Autodesk Inventor part; units mm, degrees
(part 6 of 9)
sketch "Sketch39" plane through (0, 0, 0) normal (1, 0, 0) x (0, 0, -1)
  line L0 (-85.3603, 16.259) -> (-85.3603, 6.734)
  arc A0 (-90.1228, 1.9715) -> (-85.3603, 6.734) centre (-90.1228, 6.734) ccw
  line L1 (-90.1228, 1.9715) -> (-121.8728, 1.9715)
  arc A1 (-126.6353, 6.734) -> (-121.8728, 1.9715) centre (-121.8728, 6.734) ccw
  line L2 (-126.6353, 6.734) -> (-126.6353, 16.259)
  line L3 (-126.6353, 16.259) -> (-132.3503, 16.259)
  arc A2 (-132.3503, 22.609) -> (-132.3503, 16.259) centre (-132.3503, 19.434) ccw
  line L4 (-132.3503, 22.609) -> (-126.6353, 22.609)
  line L5 (-126.6353, 22.609) -> (-126.6353, 32.134)
  arc A3 (-121.8728, 36.8965) -> (-126.6353, 32.134) centre (-121.8728, 32.134) ccw
  line L6 (-121.8728, 36.8965) -> (-90.1228, 36.8965)
  arc A4 (-85.3603, 32.134) -> (-90.1228, 36.8965) centre (-90.1228, 32.134) ccw
  line L7 (-85.3603, 32.134) -> (-85.3603, 22.609)
  line L8 (-85.3603, 22.609) -> (-79.6453, 22.609)
  arc A5 (-79.6453, 16.259) -> (-79.6453, 22.609) centre (-79.6453, 19.434) ccw
  line L9 (-79.6453, 16.259) -> (-85.3603, 16.259)
  line L10 (-121.8728, 6.734) -> (-90.1228, 6.734)
  line L11 (-90.1228, 6.734) -> (-90.1228, 32.134)
  line L12 (-90.1228, 32.134) -> (-121.8728, 32.134)
  line L13 (-121.8728, 32.134) -> (-121.8728, 6.734)
  line L14 (-121.8728, 6.734) -> (-90.1228, 32.134) construction
  line L15 (-90.1228, 6.734) -> (-121.8728, 32.134) construction
  line L16 (-131.3978, 57.3308) -> (-80.5978, 57.3308)
  line L17 (-105.9978, 19.434) -> (-105.9978, 57.3308)
  line L18 (-105.9978, -16.3292) -> (-105.9978, 19.434)
  line L19 (-112.3478, -16.3292) -> (-99.6478, -16.3292)
  circle A6 centre (-112.3478, -16.3292) radius 2.5527
  circle A7 centre (-99.6478, -16.3292) radius 2.5527
  circle A8 centre (-80.5978, 57.3308) radius 2.5527
  circle A9 centre (-131.3978, 57.3308) radius 2.5527
  line L20 (-112.3478, -13.7765) -> (-99.6478, -13.7765)
  line L21 (-99.6478, -18.8819) -> (-112.3478, -18.8819)
  line L22 (-131.3978, 59.8835) -> (-80.5978, 59.8835)
  line L23 (-80.5978, 54.7781) -> (-131.3978, 54.7781)
  arc A10 (-196.307, 76.2) -> (-199.482, 73.025) centre (-196.307, 73.025) ccw projected
  line L24 (-199.482, 73.025) -> (-199.482, -252.424) projected
  arc A11 (-199.482, -252.424) -> (-196.307, -255.599) centre (-196.307, -252.424) ccw projected
  line L25 (-196.307, -255.599) -> (147.8383, -255.599) projected
  arc A12 (147.8383, -255.599) -> (150.6952, -253.8092) centre (147.8383, -252.424) ccw projected
  line L26 (194.4526, -163.563) -> (150.6952, -253.8092) projected
  arc A13 (194.8736, -162.9119) -> (194.4526, -163.563) centre (197.3095, -164.9483) ccw projected
  arc A14 (194.8736, -162.9119) -> (235.5329, 95.0804) centre (0, 0) ccw projected
  arc A15 (235.5329, 95.0804) -> (218.389, 101.8364) centre (223.7562, 90.3263) ccw projected
  line L27 (218.389, 101.8364) -> (173.6183, 80.9596) projected
  arc A16 (152.1493, 76.2) -> (173.6183, 80.9596) centre (152.1493, 127) ccw projected
  line L28 (152.1493, 76.2) -> (-196.307, 76.2) projected
  arc A17 (-166.8187, -7.1514) -> (-170.0188, -10.965) centre (-168.4187, -9.0582) ccw projected
  arc A18 (-166.8187, -7.1514) -> (-135.2171, -21.8874) centre (-123.52, 44.45) ccw projected
  arc A19 (-136.0816, -26.7902) -> (-135.2171, -21.8874) centre (-135.6494, -24.3388) ccw projected
  arc A20 (-170.0188, -10.965) -> (-136.0816, -26.7902) centre (-123.52, 44.45) ccw projected
  circle A21 centre (-123.52, 44.45) radius 2.4892 projected
  line L29 (-117.9165, 59.8835) -> (-80.5978, 59.8835) projected
  arc A22 (-80.5978, 54.7781) -> (-80.5978, 59.8835) centre (-80.5978, 57.3308) ccw projected
  line L30 (-80.5978, 54.7781) -> (-123.0219, 54.7781) projected
  line L31 (-123.0219, 54.7781) -> (-117.9165, 59.8835) projected
  circle A23 centre (-11.1125, -19.2474) radius 2.2479 projected
  circle A24 centre (-11.1125, 19.2474) radius 2.2479 projected
  circle A25 centre (22.225, 0) radius 2.2479 projected
  circle A26 centre (11.1125, 19.2474) radius 2.2479 projected
  circle A27 centre (-22.225, 0) radius 2.2479 projected
  circle A28 centre (11.1125, -19.2474) radius 2.2479 projected
  line L32 (-112.3478, -13.7765) -> (-99.6478, -13.7765) projected
  arc A29 (-99.6478, -18.8819) -> (-99.6478, -13.7765) centre (-99.6478, -16.3292) ccw projected
  line L33 (-99.6478, -18.8819) -> (-112.3478, -18.8819) projected
  arc A30 (-112.3478, -13.7765) -> (-112.3478, -18.8819) centre (-112.3478, -16.3292) ccw projected
  circle A31 centre (-58.8554, 19.434) radius 2.4892 projected
  circle A32 centre (-76.4174, -178.6042) radius 13.335 projected
  circle A33 centre (-187.1176, -166.8269) radius 2.4892 projected
  circle A34 centre (-174.2102, -166.8866) radius 2.4892 projected
  circle A35 centre (-167.2175, -120.5501) radius 2.4892 projected
  circle A36 centre (-180.1195, -116.9252) radius 2.4892 projected
  circle A37 centre (-193.0957, -120.1058) radius 2.4892 projected
  circle A38 centre (-186.8225, -117.6771) radius 2.4892 projected
  circle A39 centre (-173.4354, -117.9041) radius 2.4892 projected
  circle A40 centre (-168.1768, -164.3742) radius 2.4892 projected
  circle A41 centre (-180.6733, -167.7222) radius 2.4892 projected
  circle A42 centre (-193.0957, -164.2646) radius 2.4892 projected
  arc A43 (-177.4857, -133.2108) -> (-183.7867, -151.2692) centre (-180.6362, -142.24) ccw projected
  arc A44 (-183.3071, -151.4366) -> (-177.0061, -133.3781) centre (-180.1566, -142.4074) ccw projected
  circle A45 centre (-85.7798, -94.9817) radius 2.4892 projected
  circle A46 centre (-110.3931, -99.2933) radius 2.4892 projected
  circle A47 centre (-101.8395, -50.0579) radius 2.4892 projected
  circle A48 centre (-124.2369, -62.8574) radius 2.4892 projected
  circle A49 centre (-110.6604, -51.6228) radius 2.4892 projected
  circle A50 centre (-93.2858, -99.3592) radius 2.4892 projected
  circle A51 centre (-116.932, -39.699) radius 2.5527 projected
  circle A52 centre (-118.4334, -56.0666) radius 2.4892 projected
  circle A53 centre (-93.0185, -51.5569) radius 2.4892 projected
  circle A54 centre (-101.8395, -100.8579) radius 2.4892 projected
  circle A55 centre (-80.2428, -88.2574) radius 2.4892 projected
  arc A56 (-99.4903, -84.728) -> (-104.0551, -66.155) centre (-101.7058, -75.4251) ccw projected
  arc A57 (-99.6119, -84.758) -> (-99.4903, -84.728) centre (-101.8395, -75.4579) ccw projected
  arc A58 (-99.7334, -84.7881) -> (-99.6119, -84.758) centre (-101.9731, -75.491) ccw projected
  arc A59 (-99.8547, -84.8183) -> (-99.7334, -84.7881) centre (-102.1066, -75.5241) ccw projected
  arc A60 (-104.4917, -66.2632) -> (-99.8547, -84.8183) centre (-102.2399, -75.5574) ccw projected
  arc A61 (-104.3463, -66.227) -> (-104.4917, -66.2632) centre (-102.1066, -75.5241) ccw projected
  arc A62 (-104.2008, -66.1909) -> (-104.3463, -66.227) centre (-101.9731, -75.491) ccw projected
  arc A63 (-104.0551, -66.155) -> (-104.2008, -66.1909) centre (-101.8395, -75.4579) ccw projected
  circle A64 centre (239.2356, -31.496) radius 3.3782 projected
  circle A65 centre (223.7295, 90.3926) radius 3.3782 projected
  circle A66 centre (239.2356, 31.496) radius 3.3782 projected
  circle A67 centre (221.404, -95.9477) radius 3.3782 projected
  line L34 (149.831, -89.2272) -> (89.9434, -38.9755) projected
  arc A68 (88.9, -36.7379) -> (89.9434, -38.9755) centre (91.821, -36.7379) ccw projected
  line L35 (88.9, -36.7379) -> (88.9, -15.621) projected
  arc A69 (91.821, -12.7) -> (88.9, -15.621) centre (91.821, -15.621) ccw projected
  line L36 (91.821, -12.7) -> (174.1799, -12.7) projected
  arc A70 (177.0893, -15.8819) -> (174.1799, -12.7) centre (174.1799, -15.621) ccw projected
  arc A71 (154.2425, -88.4425) -> (177.0893, -15.8819) centre (0, 0) ccw projected
  arc A72 (149.831, -89.2272) -> (154.2425, -88.4425) centre (151.7086, -86.9895) ccw projected
  line L37 (88.9, -0.254) -> (88.9, 0.254) projected
  arc A73 (91.821, 3.175) -> (88.9, 0.254) centre (91.821, 0.254) ccw projected
  line L38 (91.821, 3.175) -> (174.4218, 3.175) projected
  arc A74 (177.3428, 0.254) -> (174.4218, 3.175) centre (174.4218, 0.254) ccw projected
  line L39 (177.3428, 0.254) -> (177.3428, -0.254) projected
  arc A75 (174.4218, -3.175) -> (177.3428, -0.254) centre (174.4218, -0.254) ccw projected
  line L40 (174.4218, -3.175) -> (91.821, -3.175) projected
  arc A76 (88.9, -0.254) -> (91.821, -3.175) centre (91.821, -0.254) ccw projected
  arc A77 (177.0893, 15.8819) -> (169.6939, 53.0738) centre (0, 0) ccw projected
  arc A78 (174.1799, 12.7) -> (177.0893, 15.8819) centre (174.1799, 15.621) ccw projected
  line L41 (174.1799, 12.7) -> (91.821, 12.7) projected
  arc A79 (88.9, 15.621) -> (91.821, 12.7) centre (91.821, 15.621) ccw projected
  line L42 (88.9, 15.621) -> (88.9, 17.1891) projected
  arc A80 (90.5865, 19.8364) -> (88.9, 17.1891) centre (91.821, 17.1891) ccw projected
  line L43 (90.5865, 19.8364) -> (165.6716, 54.8492) projected
  arc A81 (169.6939, 53.0738) -> (165.6716, 54.8492) centre (166.9061, 52.2019) ccw projected
  arc A82 (180.8991, -105.7674) -> (203.0448, 51.8076) centre (0, 0) ccw projected
  arc A83 (204.8485, 54.889) -> (203.0448, 51.8076) centre (205.5059, 52.4355) ccw projected
  line L44 (204.8485, 54.889) -> (206.0753, 55.2177) projected
  arc A84 (209.1938, 53.3924) -> (206.0753, 55.2177) centre (206.7327, 52.7643) ccw projected
  arc A85 (186.3731, -108.9857) -> (209.1938, 53.3924) centre (0, 0) ccw projected
  arc A86 (182.8723, -109.8807) -> (186.3731, -108.9857) centre (184.1805, -107.7035) ccw projected
  line L45 (182.8723, -109.8807) -> (181.7836, -109.2266) projected
  arc A87 (180.8991, -105.7674) -> (181.7836, -109.2266) centre (183.0918, -107.0494) ccw projected
  arc A88 (159.1231, -92.6879) -> (178.5072, 45.237) centre (0, 0) ccw projected
  arc A89 (180.312, 48.3145) -> (178.5072, 45.237) centre (180.9694, 45.861) ccw projected
  line L46 (180.312, 48.3145) -> (181.5388, 48.6432) projected
  arc A90 (184.6584, 46.8139) -> (181.5388, 48.6432) centre (182.1962, 46.1897) ccw projected
  arc A91 (164.6013, -95.8992) -> (184.6584, 46.8139) centre (0, 0) ccw projected
  arc A92 (161.0985, -96.7977) -> (164.6013, -95.8992) centre (162.4067, -94.6205) ccw projected
  line L47 (161.0985, -96.7977) -> (160.0098, -96.1436) projected
  arc A93 (159.1231, -92.6879) -> (160.0098, -96.1436) centre (161.3179, -93.9664) ccw projected
  line L48 (171.9854, -103.3393) -> (170.8967, -102.6851) projected
  arc A94 (170.0112, -99.2275) -> (170.8967, -102.6851) centre (172.2049, -100.5079) ccw projected
  arc A95 (170.0112, -99.2275) -> (190.7761, 48.5222) centre (0, 0) ccw projected
  arc A96 (192.5803, 51.6017) -> (190.7761, 48.5222) centre (193.2377, 49.1483) ccw projected
  line L49 (192.5803, 51.6017) -> (193.8071, 51.9305) projected
  arc A97 (196.9261, 50.1033) -> (193.8071, 51.9305) centre (194.4645, 49.477) ccw projected
  arc A98 (175.4872, -102.4426) -> (196.9261, 50.1033) centre (0, 0) ccw projected
  arc A99 (171.9854, -103.3393) -> (175.4872, -102.4426) centre (173.2936, -101.1621) ccw projected
  circle A100 centre (187.962, 68.4126) radius 2.5527 projected
  circle A101 centre (0, 0) radius 13.335 projected
  circle A102 centre (160.7915, -118.9794) radius 2.5527 projected
  circle A103 centre (145.0649, -113.4346) radius 2.5527 projected
  circle A104 centre (122.2368, -242.899) radius 2.5527 projected
  circle A105 centre (70.3186, -242.899) radius 2.5527 projected
  circle A106 centre (97.9437, -242.899) radius 2.5527 projected
  circle A107 centre (145.0649, -242.899) radius 2.5527 projected
  circle A108 centre (-116.932, -242.899) radius 2.5527 projected
  circle A109 centre (-116.932, -179.399) radius 2.5527 projected
  circle A110 centre (-148.682, -179.399) radius 2.5527 projected
  circle A111 centre (-186.782, -39.699) radius 2.5527 projected
  circle A112 centre (-186.782, -242.899) radius 2.5527 projected
  circle A113 centre (67.218, 63.5) radius 2.5527 projected
  circle A114 centre (-59.782, 63.5) radius 2.5527 projected
  circle A115 centre (-8.982, 63.5) radius 2.5527 projected
  circle A116 centre (143.418, 63.5) radius 2.5527 projected
  circle A117 centre (-186.782, -179.399) radius 2.5527 projected
  circle A118 centre (-148.682, -39.699) radius 2.5527 projected
  circle A119 centre (-148.682, -242.899) radius 2.5527 projected
  arc A120 (-82.1853, 16.259) -> (-85.3603, 13.084) centre (-82.1853, 13.084) ccw projected
  line L50 (-85.3603, 13.084) -> (-85.3603, 6.734) projected
  arc A121 (-90.1228, 1.9715) -> (-85.3603, 6.734) centre (-90.1228, 6.734) ccw projected
  line L51 (-90.1228, 1.9715) -> (-121.8728, 1.9715) projected
  arc A122 (-126.6353, 6.734) -> (-121.8728, 1.9715) centre (-121.8728, 6.734) ccw projected
  line L52 (-126.6353, 6.734) -> (-126.6353, 13.084) projected
  arc A123 (-126.6353, 13.084) -> (-129.8103, 16.259) centre (-129.8103, 13.084) ccw projected
  line L53 (-129.8103, 16.259) -> (-132.3503, 16.259) projected
  arc A124 (-132.3503, 22.609) -> (-132.3503, 16.259) centre (-132.3503, 19.434) ccw projected
  line L54 (-132.3503, 22.609) -> (-129.8103, 22.609) projected
  arc A125 (-129.8103, 22.609) -> (-126.6353, 25.784) centre (-129.8103, 25.784) ccw projected
  line L55 (-126.6353, 25.784) -> (-126.6353, 32.134) projected
  arc A126 (-121.8728, 36.8965) -> (-126.6353, 32.134) centre (-121.8728, 32.134) ccw projected
  line L56 (-121.8728, 36.8965) -> (-90.1228, 36.8965) projected
  arc A127 (-85.3603, 32.134) -> (-90.1228, 36.8965) centre (-90.1228, 32.134) ccw projected
  line L57 (-85.3603, 32.134) -> (-85.3603, 25.784) projected
  arc A128 (-85.3603, 25.784) -> (-82.1853, 22.609) centre (-82.1853, 25.784) ccw projected
  line L58 (-82.1853, 22.609) -> (-79.6453, 22.609) projected
  arc A129 (-79.6453, 16.259) -> (-79.6453, 22.609) centre (-79.6453, 19.434) ccw projected
  line L59 (-79.6453, 16.259) -> (-82.1853, 16.259) projected
  line L60 (-121.8728, 32.134) -> (-90.1228, 6.734)
  line L61 (-90.1228, 32.134) -> (-121.8728, 6.734)
  arc A130 (-90.1228, 1.9715) -> (-85.3603, 6.734) centre (-90.1228, 6.734) ccw projected
  line L62 (-121.8728, 36.8965) -> (-90.1228, 36.8965) projected
  line L63 (-85.3603, 32.134) -> (-85.3603, 25.784) projected
  line L64 (-126.6353, 6.734) -> (-126.6353, 13.084) projected
  arc A131 (-85.3603, 32.134) -> (-90.1228, 36.8965) centre (-90.1228, 32.134) ccw projected
  arc A132 (-132.3503, 22.609) -> (-132.3503, 16.259) centre (-132.3503, 19.434) ccw projected
  line L65 (-132.3503, 22.609) -> (-129.8103, 22.609) projected
  line L66 (-129.8103, 16.259) -> (-132.3503, 16.259) projected
  line L67 (-177.4857, -133.2108) -> (-177.0061, -133.3781) projected
  line L68 (-183.3071, -151.4366) -> (-183.7867, -151.2692) projected
  point P0 (-105.9978, 19.434)
  dimension "d863" = 50.8
  dimension "d864" = 12.7
  dimension "d865" = 5.1054
  dimension "d866" = 35.7632
  dimension "d867" = 37.8968
  constraints: 52 end point, 21 point on circle, 10 centre point, 10 coincident, 10 collinear, 10 equal radius, 10 midpoint, 7 tangent, 4 horizontal, 2 parallel, 2 point on line, 2 vertical, 1 perpendicular
  measures "d863" distance of L16.end L16.start
  measures "d864" distance of L19.start L19.end
  measures "d865" diameter of A6
  measures "d866" distance from line of point (-105.998, 19.434) L19
  measures "d867" distance from line of L17.start L16
extrude "Extrusion22" cut sketch "Sketch39" against normal through all contours A9 L22 L31 L16 | A9 | L16 L31 L23 A9 | L31 L22 A8 L16 | L16 L17 L23 L31 | L16 A8 L23 L17 | A8
sketch "Sketch41" plane through (0, 0, 0) normal (1, 0, 0) x (0, 0, -1)
  arc A0 (-104.4917, -66.2632) -> (-99.8547, -84.8183) centre (-102.2399, -75.5574) ccw projected
  arc A1 (-99.4903, -84.728) -> (-104.0551, -66.155) centre (-101.7058, -75.4251) ccw projected
  circle A2 centre (-76.4174, -178.6042) radius 13.335 projected
  arc A3 (-99.4294, -84.7133) -> (-99.9153, -84.8337) centre (-76.4174, -178.6042) ccw
  arc A4 (-99.4294, -84.7133) -> (-99.9153, -84.8337) centre (-76.4174, -178.6042) ccw
  arc A5 (-103.9823, -66.1369) -> (-104.5644, -66.2812) centre (-76.4174, -178.6042) ccw
  line L0 (-99.9153, -84.8337) -> (-104.5644, -66.2812)
  line L1 (-99.4294, -84.7133) -> (-103.9823, -66.1369)
  point P0 (0, 0)
  constraints: 10 point on circle, 4 end point, 3 centre point, 3 coincident, 3 tangent
extrude "Extrusion24" cut sketch "Sketch41" against normal through all contours A5 A1 L1 A3 A0 L0
sketch "Sketch43" plane through (0, 0, 0) normal (1, 0, 0) x (0, 0, -1)
  arc A0 (-103.9823, -66.1369) -> (-104.5644, -66.2812) centre (-76.4174, -178.6042) ccw projected
  arc A1 (-99.4294, -84.7133) -> (-103.9823, -66.1369) centre (-101.7058, -75.4251) ccw projected
  arc A2 (-99.4294, -84.7133) -> (-99.9153, -84.8337) centre (-76.4174, -178.6042) ccw projected
  arc A3 (-104.5644, -66.2812) -> (-99.9153, -84.8337) centre (-102.2399, -75.5574) ccw projected
  arc A4 (-82.1853, 16.259) -> (-85.3603, 13.084) centre (-82.1853, 13.084) ccw projected
  line L0 (-85.3603, 13.084) -> (-85.3603, 6.734) projected
  arc A5 (-90.1228, 1.9715) -> (-85.3603, 6.734) centre (-90.1228, 6.734) ccw projected
  line L1 (-90.1228, 1.9715) -> (-121.8728, 1.9715) projected
  arc A6 (-126.6353, 6.734) -> (-121.8728, 1.9715) centre (-121.8728, 6.734) ccw projected
  line L2 (-126.6353, 6.734) -> (-126.6353, 13.084) projected
  arc A7 (-126.6353, 13.084) -> (-129.8103, 16.259) centre (-129.8103, 13.084) ccw projected
  line L3 (-129.8103, 16.259) -> (-132.3503, 16.259) projected
  arc A8 (-132.3503, 22.609) -> (-132.3503, 16.259) centre (-132.3503, 19.434) ccw projected
  line L4 (-132.3503, 22.609) -> (-129.8103, 22.609) projected
  arc A9 (-129.8103, 22.609) -> (-126.6353, 25.784) centre (-129.8103, 25.784) ccw projected
  line L5 (-126.6353, 25.784) -> (-126.6353, 32.134) projected
  arc A10 (-121.8728, 36.8965) -> (-126.6353, 32.134) centre (-121.8728, 32.134) ccw projected
  line L6 (-121.8728, 36.8965) -> (-90.1228, 36.8965) projected
  arc A11 (-85.3603, 32.134) -> (-90.1228, 36.8965) centre (-90.1228, 32.134) ccw projected
  line L7 (-85.3603, 32.134) -> (-85.3603, 25.784) projected
  arc A12 (-85.3603, 25.784) -> (-82.1853, 22.609) centre (-82.1853, 25.784) ccw projected
  line L8 (-82.1853, 22.609) -> (-79.6453, 22.609) projected
  arc A13 (-79.6453, 16.259) -> (-79.6453, 22.609) centre (-79.6453, 19.434) ccw projected
  line L9 (-79.6453, 16.259) -> (-82.1853, 16.259) projected
  line L10 (-112.3478, -13.7765) -> (-99.6478, -13.7765) projected
  arc A14 (-99.6478, -18.8819) -> (-99.6478, -13.7765) centre (-99.6478, -16.3292) ccw projected
  line L11 (-99.6478, -18.8819) -> (-112.3478, -18.8819) projected
  arc A15 (-112.3478, -13.7765) -> (-112.3478, -18.8819) centre (-112.3478, -16.3292) ccw projected
  circle A16 centre (-58.8554, 19.434) radius 2.4892 projected
  line L12 (-177.4857, -133.2108) -> (-177.0061, -133.3781) projected
  arc A17 (-183.3071, -151.4366) -> (-177.0061, -133.3781) centre (-180.1566, -142.4074) ccw projected
  line L13 (-183.3071, -151.4366) -> (-183.7867, -151.2692) projected
  arc A18 (-177.4857, -133.2108) -> (-183.7867, -151.2692) centre (-180.6362, -142.24) ccw projected
  circle A19 centre (-76.4174, -178.6042) radius 13.335 projected
  circle A20 centre (-187.1176, -166.8269) radius 2.4892 projected
  circle A21 centre (-174.2102, -166.8866) radius 2.4892 projected
  circle A22 centre (-167.2175, -120.5501) radius 2.4892 projected
  circle A23 centre (-180.1195, -116.9252) radius 2.4892 projected
  circle A24 centre (-193.0957, -120.1058) radius 2.4892 projected
  circle A25 centre (-186.8225, -117.6771) radius 2.4892 projected
  circle A26 centre (-173.4354, -117.9041) radius 2.4892 projected
  circle A27 centre (-168.1768, -164.3742) radius 2.4892 projected
  circle A28 centre (-180.6733, -167.7222) radius 2.4892 projected
  circle A29 centre (-193.0957, -164.2646) radius 2.4892 projected
  circle A30 centre (-85.7798, -94.9817) radius 2.4892 projected
  circle A31 centre (-110.3931, -99.2933) radius 2.4892 projected
  circle A32 centre (-101.8395, -50.0579) radius 2.4892 projected
  circle A33 centre (-124.2369, -62.8574) radius 2.4892 projected
  circle A34 centre (-110.6604, -51.6228) radius 2.4892 projected
  circle A35 centre (-93.2858, -99.3592) radius 2.4892 projected
  circle A36 centre (-118.4334, -56.0666) radius 2.4892 projected
  circle A37 centre (-93.0185, -51.5569) radius 2.4892 projected
  circle A38 centre (-101.8395, -100.8579) radius 2.4892 projected
  circle A39 centre (-80.2428, -88.2574) radius 2.4892 projected
  circle A40 centre (239.2356, -31.496) radius 3.3782 projected
  circle A41 centre (223.7295, 90.3926) radius 3.3782 projected
  circle A42 centre (239.2356, 31.496) radius 3.3782 projected
  circle A43 centre (221.404, -95.9477) radius 3.3782 projected
  line L14 (149.831, -89.2272) -> (89.9434, -38.9755) projected
  arc A44 (88.9, -36.7379) -> (89.9434, -38.9755) centre (91.821, -36.7379) ccw projected
  line L15 (88.9, -36.7379) -> (88.9, -15.621) projected
  arc A45 (91.821, -12.7) -> (88.9, -15.621) centre (91.821, -15.621) ccw projected
  line L16 (91.821, -12.7) -> (174.1799, -12.7) projected
  arc A46 (177.0893, -15.8819) -> (174.1799, -12.7) centre (174.1799, -15.621) ccw projected
  arc A47 (154.2425, -88.4425) -> (177.0893, -15.8819) centre (0, 0) ccw projected
  arc A48 (149.831, -89.2272) -> (154.2425, -88.4425) centre (151.7086, -86.9895) ccw projected
  line L17 (88.9, -0.254) -> (88.9, 0.254) projected
  arc A49 (91.821, 3.175) -> (88.9, 0.254) centre (91.821, 0.254) ccw projected
  line L18 (91.821, 3.175) -> (174.4218, 3.175) projected
  arc A50 (177.3428, 0.254) -> (174.4218, 3.175) centre (174.4218, 0.254) ccw projected
  line L19 (177.3428, 0.254) -> (177.3428, -0.254) projected
  arc A51 (174.4218, -3.175) -> (177.3428, -0.254) centre (174.4218, -0.254) ccw projected
  line L20 (174.4218, -3.175) -> (91.821, -3.175) projected
  arc A52 (88.9, -0.254) -> (91.821, -3.175) centre (91.821, -0.254) ccw projected
  arc A53 (177.0893, 15.8819) -> (169.6939, 53.0738) centre (0, 0) ccw projected
  arc A54 (174.1799, 12.7) -> (177.0893, 15.8819) centre (174.1799, 15.621) ccw projected
  line L21 (174.1799, 12.7) -> (91.821, 12.7) projected
  arc A55 (88.9, 15.621) -> (91.821, 12.7) centre (91.821, 15.621) ccw projected
  line L22 (88.9, 15.621) -> (88.9, 17.1891) projected
  arc A56 (90.5865, 19.8364) -> (88.9, 17.1891) centre (91.821, 17.1891) ccw projected
  line L23 (90.5865, 19.8364) -> (165.6716, 54.8492) projected
  arc A57 (169.6939, 53.0738) -> (165.6716, 54.8492) centre (166.9061, 52.2019) ccw projected
  arc A58 (180.8991, -105.7674) -> (203.0448, 51.8076) centre (0, 0) ccw projected
  arc A59 (204.8485, 54.889) -> (203.0448, 51.8076) centre (205.5059, 52.4355) ccw projected
  line L24 (204.8485, 54.889) -> (206.0753, 55.2177) projected
  arc A60 (209.1938, 53.3924) -> (206.0753, 55.2177) centre (206.7327, 52.7643) ccw projected
  arc A61 (186.3731, -108.9857) -> (209.1938, 53.3924) centre (0, 0) ccw projected
  arc A62 (182.8723, -109.8807) -> (186.3731, -108.9857) centre (184.1805, -107.7035) ccw projected
  line L25 (182.8723, -109.8807) -> (181.7836, -109.2266) projected
  arc A63 (180.8991, -105.7674) -> (181.7836, -109.2266) centre (183.0918, -107.0494) ccw projected
  arc A64 (159.1231, -92.6879) -> (178.5072, 45.237) centre (0, 0) ccw projected
  arc A65 (180.312, 48.3145) -> (178.5072, 45.237) centre (180.9694, 45.861) ccw projected
  line L26 (180.312, 48.3145) -> (181.5388, 48.6432) projected
  arc A66 (184.6584, 46.8139) -> (181.5388, 48.6432) centre (182.1962, 46.1897) ccw projected
  arc A67 (164.6013, -95.8992) -> (184.6584, 46.8139) centre (0, 0) ccw projected
  arc A68 (161.0985, -96.7977) -> (164.6013, -95.8992) centre (162.4067, -94.6205) ccw projected
  line L27 (161.0985, -96.7977) -> (160.0098, -96.1436) projected
  arc A69 (159.1231, -92.6879) -> (160.0098, -96.1436) centre (161.3179, -93.9664) ccw projected
  line L28 (171.9854, -103.3393) -> (170.8967, -102.6851) projected
  arc A70 (170.0112, -99.2275) -> (170.8967, -102.6851) centre (172.2049, -100.5079) ccw projected
  arc A71 (170.0112, -99.2275) -> (190.7761, 48.5222) centre (0, 0) ccw projected
  arc A72 (192.5803, 51.6017) -> (190.7761, 48.5222) centre (193.2377, 49.1483) ccw projected
  line L29 (192.5803, 51.6017) -> (193.8071, 51.9305) projected
  arc A73 (196.9261, 50.1033) -> (193.8071, 51.9305) centre (194.4645, 49.477) ccw projected
  arc A74 (175.4872, -102.4426) -> (196.9261, 50.1033) centre (0, 0) ccw projected
  arc A75 (171.9854, -103.3393) -> (175.4872, -102.4426) centre (173.2936, -101.1621) ccw projected
  circle A76 centre (187.962, 68.4126) radius 2.5527 projected
  circle A77 centre (0, 0) radius 13.335 projected
  circle A78 centre (160.7915, -118.9794) radius 2.5527 projected
  circle A79 centre (145.0649, -113.4346) radius 2.5527 projected
  circle A80 centre (122.2368, -242.899) radius 2.5527 projected
  circle A81 centre (70.3186, -242.899) radius 2.5527 projected
  circle A82 centre (97.9437, -242.899) radius 2.5527 projected
  circle A83 centre (145.0649, -242.899) radius 2.5527 projected
  circle A84 centre (-116.932, -242.899) radius 2.5527 projected
  circle A85 centre (-116.932, -179.399) radius 2.5527 projected
  circle A86 centre (-148.682, -179.399) radius 2.5527 projected
  circle A87 centre (-186.782, -39.699) radius 2.5527 projected
  circle A88 centre (-186.782, -242.899) radius 2.5527 projected
  circle A89 centre (67.218, 63.5) radius 2.5527 projected
  circle A90 centre (-59.782, 63.5) radius 2.5527 projected
  circle A91 centre (-8.982, 63.5) radius 2.5527 projected
  circle A92 centre (143.418, 63.5) radius 2.5527 projected
  circle A93 centre (-186.782, -179.399) radius 2.5527 projected
  circle A94 centre (-148.682, -39.699) radius 2.5527 projected
  circle A95 centre (-116.932, -39.699) radius 2.5527 projected
  circle A96 centre (-148.682, -242.899) radius 2.5527 projected
  circle A97 centre (11.1125, -19.2474) radius 2.2479 projected
  circle A98 centre (-22.225, 0) radius 2.2479 projected
  circle A99 centre (11.1125, 19.2474) radius 2.2479 projected
  circle A100 centre (22.225, 0) radius 2.2479 projected
  circle A101 centre (-11.1125, 19.2474) radius 2.2479 projected
  circle A102 centre (-11.1125, -19.2474) radius 2.2479 projected
  line L30 (-80.5978, 54.7781) -> (-131.3978, 54.7781) projected
  arc A103 (-131.3978, 59.8835) -> (-131.3978, 54.7781) centre (-131.3978, 57.3308) ccw projected
  line L31 (-131.3978, 59.8835) -> (-80.5978, 59.8835) projected
  arc A104 (-80.5978, 54.7781) -> (-80.5978, 59.8835) centre (-80.5978, 57.3308) ccw projected
  circle A105 centre (-123.52, 44.45) radius 2.4892 projected
  arc A106 (-166.8187, -7.1514) -> (-170.0188, -10.965) centre (-168.4187, -9.0582) ccw projected
  arc A107 (-166.8187, -7.1514) -> (-135.2171, -21.8874) centre (-123.52, 44.45) ccw projected
  arc A108 (-136.0816, -26.7902) -> (-135.2171, -21.8874) centre (-135.6494, -24.3388) ccw projected
  arc A109 (-170.0188, -10.965) -> (-136.0816, -26.7902) centre (-123.52, 44.45) ccw projected
  arc A110 (-196.307, 76.2) -> (-199.482, 73.025) centre (-196.307, 73.025) ccw projected
  line L32 (-199.482, 73.025) -> (-199.482, -252.424) projected
  arc A111 (-199.482, -252.424) -> (-196.307, -255.599) centre (-196.307, -252.424) ccw projected
  line L33 (-196.307, -255.599) -> (147.8383, -255.599) projected
  arc A112 (147.8383, -255.599) -> (150.6952, -253.8092) centre (147.8383, -252.424) ccw projected
  line L34 (194.4526, -163.563) -> (150.6952, -253.8092) projected
  arc A113 (194.8736, -162.9119) -> (194.4526, -163.563) centre (197.3095, -164.9483) ccw projected
  arc A114 (194.8736, -162.9119) -> (235.5329, 95.0804) centre (0, 0) ccw projected
  arc A115 (235.5329, 95.0804) -> (218.389, 101.8364) centre (223.7562, 90.3263) ccw projected
  line L35 (218.389, 101.8364) -> (173.6183, 80.9596) projected
  arc A116 (152.1493, 76.2) -> (173.6183, 80.9596) centre (152.1493, 127) ccw projected
  line L36 (152.1493, 76.2) -> (-196.307, 76.2) projected
  arc A117 (-85.6539, -48.4094) -> (-88.99, -46.6745) centre (-90.1204, -52.923) ccw projected
  arc A118 (-114.689, -104.2414) -> (-85.6539, -48.4094) centre (-101.8395, -75.4579) ccw projected
  arc A119 (-118.0252, -102.5065) -> (-114.689, -104.2414) centre (-113.5587, -97.9928) ccw projected
  arc A120 (-88.99, -46.6745) -> (-118.0252, -102.5065) centre (-101.8395, -75.4579) ccw projected
  arc A121 (-84.1306, -35.1868) -> (-84.8012, -35.3982) centre (-84.3454, -35.6751) ccw projected
  arc A122 (-85.259, -35.965) -> (-84.8012, -35.3982) centre (-87.1419, -33.9761) ccw projected
  arc A123 (-87.6678, -35.0381) -> (-85.259, -35.965) centre (-86.2421, -34.9266) ccw projected
  arc A124 (-87.6275, -34.3106) -> (-87.6678, -35.0381) centre (-84.9373, -34.8245) ccw projected
  arc A125 (-87.6275, -34.3106) -> (-87.9834, -33.7042) centre (-88.1514, -34.2105) ccw projected
  arc A126 (-87.9834, -33.7042) -> (-88.7509, -33.4573) centre (-101.8395, -75.4579) ccw projected
  arc A127 (-88.7509, -33.4573) -> (-89.3936, -33.7424) centre (-88.9096, -33.9665) ccw projected
  arc A128 (-89.7851, -34.3569) -> (-89.3936, -33.7424) centre (-91.8788, -32.5913) ccw projected
  arc A129 (-92.2825, -33.7055) -> (-89.7851, -34.3569) centre (-90.8783, -33.4351) ccw projected
  arc A130 (-92.3239, -32.978) -> (-92.2825, -33.7055) centre (-89.5931, -33.1875) ccw projected
  arc A131 (-92.3239, -32.978) -> (-92.7455, -32.4154) centre (-92.8557, -32.9372) ccw projected
  arc A132 (-92.7455, -32.4154) -> (-93.5358, -32.2559) centre (-101.8395, -75.4579) ccw projected
  arc A133 (-93.5358, -32.2559) -> (-94.1425, -32.6112) centre (-93.6365, -32.7797) ccw projected
  arc A134 (-94.4627, -33.2657) -> (-94.1425, -32.6112) centre (-96.741, -31.7456) ccw projected
  arc A135 (-97.0174, -32.898) -> (-94.4627, -33.2657) centre (-95.6523, -32.472) ccw projected
  arc A136 (-97.14, -32.1797) -> (-97.0174, -32.898) centre (-94.4029, -32.0822) ccw projected
  arc A137 (-97.14, -32.1797) -> (-97.6219, -31.6678) centre (-97.673, -32.1987) ccw projected
  arc A138 (-97.6219, -31.6678) -> (-98.4251, -31.5978) centre (-101.8395, -75.4579) ccw projected
  arc A139 (-98.4251, -31.5978) -> (-98.9883, -32.0188) centre (-98.4665, -32.1296) ccw projected
  arc A140 (-99.2331, -32.7051) -> (-98.9883, -32.0188) centre (-101.6673, -31.4496) ccw projected
  arc A141 (-101.8129, -32.6257) -> (-99.2331, -32.7051) centre (-100.5041, -32.0496) ccw projected
  arc A142 (-102.0151, -31.9257) -> (-101.8129, -32.6257) centre (-99.3062, -31.5223) ccw projected
  arc A143 (-102.0151, -31.9257) -> (-102.5514, -31.4709) centre (-102.5427, -32.0042) ccw projected
  arc A144 (-102.5514, -31.4709) -> (-103.3573, -31.4913) centre (-101.8395, -75.4579) ccw projected
  arc A145 (-103.3573, -31.4913) -> (-103.8698, -31.9727) centre (-103.3389, -32.0244) ccw projected
  arc A146 (-104.0363, -32.6821) -> (-103.8698, -31.9727) centre (-106.5957, -31.7071) ccw projected
  arc A147 (-106.6088, -32.892) -> (-104.0363, -32.6821) centre (-105.3727, -32.173) ccw projected
  arc A148 (-106.8881, -32.2191) -> (-106.6088, -32.892) centre (-104.2414, -31.5149) ccw projected
  arc A149 (-106.8881, -32.2191) -> (-107.4719, -31.8272) centre (-107.4036, -32.3562) ccw projected
  arc A150 (-107.4719, -31.8272) -> (-108.2705, -31.9377) centre (-101.8395, -75.4579) ccw projected
  arc A151 (-108.2705, -31.9377) -> (-108.7259, -32.4734) centre (-108.1925, -32.4654) ccw projected
  arc A152 (-108.8119, -33.197) -> (-108.7259, -32.4734) centre (-111.4644, -32.5147) ccw projected
  arc A153 (-111.3446, -33.6937) -> (-108.8119, -33.197) centre (-110.1968, -32.8407) ccw projected
  arc A154 (-111.6976, -33.0562) -> (-111.3446, -33.6937) centre (-109.1463, -32.0601) ccw projected
  arc A155 (-111.6976, -33.0562) -> (-112.3216, -32.7321) centre (-112.1945, -33.2502) ccw projected
  arc A156 (-112.3216, -32.7321) -> (-113.1028, -32.9314) centre (-101.8395, -75.4579) ccw projected
  arc A157 (-113.1028, -32.9314) -> (-113.4953, -33.5147) centre (-112.9662, -33.447) ccw projected
  arc A158 (-113.4998, -34.2434) -> (-113.4953, -33.5147) centre (-116.212, -33.8623) ccw projected
  arc A159 (-115.961, -35.0205) -> (-113.4998, -34.2434) centre (-114.9159, -34.0444) ccw projected
  arc A160 (-116.3831, -34.4266) -> (-115.961, -35.0205) centre (-113.9594, -33.1511) ccw projected
  arc A161 (-116.3831, -34.4266) -> (-117.0394, -34.1744) centre (-116.8551, -34.675) ccw projected
  arc A162 (-117.0394, -34.1744) -> (-117.7934, -34.4599) centre (-101.8395, -75.4579) ccw projected
  arc A163 (-117.7934, -34.4599) -> (-118.1182, -35.0835) centre (-117.6, -34.957) ccw projected
  arc A164 (-118.041, -35.8081) -> (-118.1182, -35.0835) centre (-120.7788, -35.7331) ccw projected
  arc A165 (-120.3998, -36.8559) -> (-118.041, -35.8081) centre (-119.4705, -35.7689) ccw projected
  arc A166 (-120.8857, -36.3129) -> (-120.3998, -36.8559) centre (-118.6201, -34.7741) ccw projected
  arc A167 (-120.8857, -36.3129) -> (-121.5661, -36.1358) centre (-121.327, -36.6126) ccw projected
  arc A168 (-121.5661, -36.1358) -> (-122.2834, -36.5039) centre (-101.8395, -75.4579) ccw projected
  arc A169 (-122.2834, -36.5039) -> (-122.5363, -37.16) centre (-122.0356, -36.9763) ccw projected
  arc A170 (-122.3785, -37.8714) -> (-122.5363, -37.16) centre (-125.1075, -38.1034) ccw projected
  arc A171 (-124.6051, -39.1767) -> (-122.3785, -37.8714) centre (-123.8034, -37.9925) ccw projected
  arc A172 (-125.1488, -38.6915) -> (-124.6051, -39.1767) centre (-123.0697, -36.9087) ccw projected
  arc A173 (-125.1488, -38.6915) -> (-125.8448, -38.5918) centre (-125.5537, -39.0388) ccw projected
  arc A174 (-125.8448, -38.5918) -> (-126.5163, -39.0379) centre (-101.8395, -75.4579) ccw projected
  arc A175 (-126.5163, -39.0379) -> (-126.6942, -39.7181) centre (-126.2171, -39.4795) ccw projected
  arc A176 (-126.4578, -40.4073) -> (-126.6942, -39.7181) centre (-129.1436, -40.9435) ccw projected
  arc A177 (-128.5242, -41.9537) -> (-126.4578, -40.4073) centre (-127.8601, -40.6873) ccw projected
  arc A178 (-129.1188, -41.5325) -> (-128.5242, -41.9537) centre (-127.2523, -39.5281) ccw projected
  arc A179 (-129.1188, -41.5325) -> (-129.8215, -41.5113) centre (-129.4823, -41.9229) ccw projected
  arc A180 (-129.8215, -41.5113) -> (-130.4389, -42.0298) centre (-101.8395, -75.4579) ccw projected
  arc A181 (-130.4389, -42.0298) -> (-130.5395, -42.7257) centre (-130.0922, -42.4351) ccw projected
  arc A182 (-130.2274, -43.3841) -> (-130.5395, -42.7257) centre (-132.8363, -44.2176) ccw projected
  arc A183 (-132.1077, -45.1521) -> (-130.2274, -43.3841) centre (-131.5896, -43.8193) ccw projected
  arc A184 (-132.7457, -44.8002) -> (-132.1077, -45.1521) centre (-131.1154, -42.5994) ccw projected
  arc A185 (-132.7457, -44.8002) -> (-133.4464, -44.8577) centre (-133.0632, -45.2288) ccw projected
  arc A186 (-133.4464, -44.8577) -> (-134.0019, -45.4421) centre (-101.8395, -75.4579) ccw projected
  arc A187 (-134.0019, -45.4421) -> (-134.0239, -46.1449) centre (-133.6119, -45.806) ccw projected
  arc A188 (-133.64, -46.7642) -> (-134.0239, -46.1449) centre (-136.1392, -47.8845) ccw projected
  arc A189 (-135.3105, -48.7317) -> (-133.64, -46.7642) centre (-134.9449, -47.3492) ccw projected
  arc A190 (-135.9839, -48.4533) -> (-135.3105, -48.7317) centre (-134.6103, -46.0839) ccw projected
  arc A191 (-135.9839, -48.4533) -> (-136.6738, -48.589) centre (-136.2514, -48.9148) ccw projected
  arc A192 (-136.6738, -48.589) -> (-137.1604, -49.2319) centre (-101.8395, -75.4579) ccw projected
  arc A193 (-137.1604, -49.2319) -> (-137.1035, -49.9327) centre (-136.7321, -49.5499) ccw projected
  arc A194 (-136.6528, -50.5051) -> (-137.1035, -49.9327) centre (-139.0108, -51.8983) ccw projected
  arc A195 (-138.0925, -52.6473) -> (-136.6528, -50.5051) centre (-137.884, -51.2325) ccw projected
  arc A196 (-138.7928, -52.4461) -> (-138.0925, -52.6473) centre (-137.6931, -49.9377) ccw projected
  arc A197 (-138.7928, -52.4461) -> (-139.4631, -52.6581) centre (-139.007, -52.9346) ccw projected
  arc A198 (-139.4631, -52.6581) -> (-139.8746, -53.3515) centre (-101.8395, -75.4579) ccw projected
  arc A199 (-139.8746, -53.3515) -> (-139.7397, -54.0415) centre (-139.4135, -53.6195) ccw projected
  arc A200 (-139.2277, -54.5599) -> (-139.7397, -54.0415) centre (-141.4149, -56.2083) ccw projected
  arc A201 (-140.4185, -56.8497) -> (-139.2277, -54.5599) centre (-140.3697, -55.4205) ccw projected
  arc A202 (-141.137, -56.7282) -> (-140.4185, -56.8497) centre (-140.325, -54.1125) ccw projected
  arc A203 (-141.137, -56.7282) -> (-141.7793, -57.014) centre (-141.2951, -57.2376) ccw projected
  arc A204 (-141.7793, -57.014) -> (-142.1106, -57.749) centre (-101.8395, -75.4579) ccw projected
  arc A205 (-142.1106, -57.749) -> (-141.8993, -58.4196) centre (-141.6224, -57.9638) ccw projected
  arc A206 (-141.3324, -58.8774) -> (-141.8993, -58.4196) centre (-143.3214, -60.7603) ccw projected
  arc A207 (-142.2594, -61.2862) -> (-141.3324, -58.8774) centre (-142.3709, -59.8605) ccw projected
  arc A208 (-142.9869, -61.2459) -> (-142.2594, -61.2862) centre (-142.473, -58.5557) ccw projected
  arc A209 (-142.9869, -61.2459) -> (-143.5933, -61.6018) centre (-143.087, -61.7698) ccw projected
  arc A210 (-143.5933, -61.6018) -> (-143.8402, -62.3693) centre (-101.8395, -75.4579) ccw projected
  arc A211 (-143.8402, -62.3693) -> (-143.5551, -63.012) centre (-143.3309, -62.528) ccw projected
  arc A212 (-142.9405, -63.4035) -> (-143.5551, -63.012) centre (-144.7061, -65.4972) ccw projected
  arc A213 (-143.592, -65.9009) -> (-142.9405, -63.4035) centre (-143.8624, -64.4967) ccw projected
  arc A214 (-144.3194, -65.9423) -> (-143.592, -65.9009) centre (-144.1099, -63.2115) ccw projected
  arc A215 (-144.3194, -65.9423) -> (-144.8821, -66.3639) centre (-144.3602, -66.4741) ccw projected
  arc A216 (-144.8821, -66.3639) -> (-145.0416, -67.1542) centre (-101.8395, -75.4579) ccw projected
  arc A217 (-145.0416, -67.1542) -> (-144.6863, -67.7609) centre (-144.5177, -67.2549) ccw projected
  arc A218 (-144.0318, -68.0811) -> (-144.6863, -67.7609) centre (-145.5519, -70.3594) ccw projected
  arc A219 (-144.3995, -70.6358) -> (-144.0318, -68.0811) centre (-144.8255, -69.2707) ccw projected
  arc A220 (-145.1178, -70.7584) -> (-144.3995, -70.6358) centre (-145.2153, -68.0213) ccw projected
  arc A221 (-145.1178, -70.7584) -> (-145.6297, -71.2403) centre (-145.0988, -71.2914) ccw projected
  arc A222 (-145.6297, -71.2403) -> (-145.6996, -72.0435) centre (-101.8395, -75.4579) ccw projected
  arc A223 (-145.6996, -72.0435) -> (-145.2787, -72.6067) centre (-145.1678, -72.0849) ccw projected
  arc A224 (-144.5924, -72.8515) -> (-145.2787, -72.6067) centre (-145.8479, -75.2857) ccw projected
  arc A225 (-144.6718, -75.4313) -> (-144.5924, -72.8515) centre (-145.2479, -74.1225) ccw projected
  arc A226 (-145.3718, -75.6336) -> (-144.6718, -75.4313) centre (-145.7752, -72.9246) ccw projected
  arc A227 (-145.3718, -75.6336) -> (-145.8266, -76.1698) centre (-145.2932, -76.1611) ccw projected
  arc A228 (-145.8266, -76.1698) -> (-145.8061, -76.9757) centre (-101.8395, -75.4579) ccw projected
  arc A229 (-145.8061, -76.9757) -> (-145.3248, -77.4882) centre (-145.2731, -76.9573) ccw projected
  arc A230 (-144.6154, -77.6547) -> (-145.3248, -77.4882) centre (-145.5904, -80.2141) ccw projected
  arc A231 (-144.4054, -80.2272) -> (-144.6154, -77.6547) centre (-145.1245, -78.9911) ccw projected
  arc A232 (-145.0784, -80.5065) -> (-144.4054, -80.2272) centre (-145.7826, -77.8598) ccw projected
  arc A233 (-145.0784, -80.5065) -> (-145.4703, -81.0903) centre (-144.9413, -81.022) ccw projected
  arc A234 (-145.4703, -81.0903) -> (-145.3598, -81.8889) centre (-101.8395, -75.4579) ccw projected
  arc A235 (-145.3598, -81.8889) -> (-144.824, -82.3443) centre (-144.8321, -81.8109) ccw projected
  arc A236 (-144.1005, -82.4303) -> (-144.824, -82.3443) centre (-144.7828, -85.0828) ccw projected
  arc A237 (-143.6038, -84.9631) -> (-144.1005, -82.4303) centre (-144.4567, -83.8152) ccw projected
  arc A238 (-144.2413, -85.316) -> (-143.6038, -84.9631) centre (-145.2374, -82.7647) ccw projected
  arc A239 (-144.2413, -85.316) -> (-144.5653, -85.94) centre (-144.0473, -85.8129) ccw projected
  arc A240 (-144.5653, -85.94) -> (-144.3661, -86.7212) centre (-101.8395, -75.4579) ccw projected
  arc A241 (-144.3661, -86.7212) -> (-143.7827, -87.1137) centre (-143.8504, -86.5846) ccw projected
  arc A242 (-143.0541, -87.1182) -> (-143.7827, -87.1137) centre (-143.4351, -89.8304) ccw projected
  arc A243 (-142.277, -89.5794) -> (-143.0541, -87.1182) centre (-143.2531, -88.5343) ccw projected
  arc A244 (-142.8709, -90.0015) -> (-142.277, -89.5794) centre (-144.1464, -87.5778) ccw projected
  arc A245 (-142.8709, -90.0015) -> (-143.1231, -90.6578) centre (-142.6225, -90.4735) ccw projected
  arc A246 (-143.1231, -90.6578) -> (-142.8376, -91.4118) centre (-101.8395, -75.4579) ccw projected
  arc A247 (-142.8376, -91.4118) -> (-142.214, -91.7366) centre (-142.3405, -91.2184) ccw projected
  arc A248 (-141.4894, -91.6594) -> (-142.214, -91.7366) centre (-141.5644, -94.3972) ccw projected
  arc A249 (-140.4416, -94.0182) -> (-141.4894, -91.6594) centre (-141.5286, -93.0889) ccw projected
  arc A250 (-140.9846, -94.5041) -> (-140.4416, -94.0182) centre (-142.5234, -92.2385) ccw projected
  arc A251 (-140.9846, -94.5041) -> (-141.1616, -95.1845) centre (-140.6849, -94.9454) ccw projected
  arc A252 (-141.1616, -95.1845) -> (-140.7935, -95.9018) centre (-101.8395, -75.4579) ccw projected
  arc A253 (-140.7935, -95.9018) -> (-140.1375, -96.1547) centre (-140.3212, -95.654) ccw projected
  arc A254 (-139.4261, -95.997) -> (-140.1375, -96.1547) centre (-139.1941, -98.7259) ccw projected
  arc A255 (-138.1208, -98.2235) -> (-139.4261, -95.997) centre (-139.305, -97.4218) ccw projected
  arc A256 (-138.6059, -98.7672) -> (-138.1208, -98.2235) centre (-140.3888, -96.6881) ccw projected
  arc A257 (-138.6059, -98.7672) -> (-138.7057, -99.4632) centre (-138.2587, -99.1721) ccw projected
  arc A258 (-138.7057, -99.4632) -> (-138.2596, -100.1348) centre (-101.8395, -75.4579) ccw projected
  arc A259 (-138.2596, -100.1348) -> (-137.5794, -100.3126) centre (-137.818, -99.8356) ccw projected
  arc A260 (-136.8901, -100.0762) -> (-137.5794, -100.3126) centre (-136.354, -102.762) ccw projected
  arc A261 (-135.3437, -102.1426) -> (-136.8901, -100.0762) centre (-136.6102, -101.4785) ccw projected
  arc A262 (-135.7649, -102.7372) -> (-135.3437, -102.1426) centre (-137.7693, -100.8707) ccw projected
  arc A263 (-135.7649, -102.7372) -> (-135.7862, -103.4399) centre (-135.3746, -103.1007) ccw projected
  arc A264 (-135.7862, -103.4399) -> (-135.2677, -104.0573) centre (-101.8395, -75.4579) ccw projected
  arc A265 (-135.2677, -104.0573) -> (-134.5718, -104.1579) centre (-134.8624, -103.7106) ccw projected
  arc A266 (-133.9134, -103.8458) -> (-134.5718, -104.1579) centre (-133.0799, -106.4547) ccw projected
  arc A267 (-132.1453, -105.7261) -> (-133.9134, -103.8458) centre (-133.4782, -105.208) ccw projected
  arc A268 (-132.4973, -106.3641) -> (-132.1453, -105.7261) centre (-134.6981, -104.7338) ccw projected
  arc A269 (-132.4973, -106.3641) -> (-132.4397, -107.0648) centre (-132.0687, -106.6816) ccw projected
  arc A270 (-132.4397, -107.0648) -> (-131.8554, -107.6203) centre (-101.8395, -75.4579) ccw projected
  arc A271 (-131.8554, -107.6203) -> (-131.1526, -107.6423) centre (-131.4914, -107.2303) ccw projected
  arc A272 (-130.5333, -107.2584) -> (-131.1526, -107.6423) centre (-129.4129, -109.7576) ccw projected
  arc A273 (-128.5658, -108.9289) -> (-130.5333, -107.2584) centre (-129.9483, -108.5633) ccw projected
  arc A274 (-128.8442, -109.6023) -> (-128.5658, -108.9289) centre (-131.2136, -108.2287) ccw projected
  arc A275 (-128.8442, -109.6023) -> (-128.7085, -110.2922) centre (-128.3827, -109.8699) ccw projected
  arc A276 (-128.7085, -110.2922) -> (-128.0656, -110.7788) centre (-101.8395, -75.4579) ccw projected
  arc A277 (-128.0656, -110.7788) -> (-127.3648, -110.722) centre (-127.7476, -110.3505) ccw projected
  arc A278 (-126.7923, -110.2712) -> (-127.3648, -110.722) centre (-125.3992, -112.6292) ccw projected
  arc A279 (-124.6502, -111.7109) -> (-126.7923, -110.2712) centre (-126.065, -111.5024) ccw projected
  arc A280 (-124.8514, -112.4112) -> (-124.6502, -111.7109) centre (-127.3598, -111.3115) ccw projected
  arc A281 (-124.8514, -112.4112) -> (-124.6393, -113.0815) centre (-124.3629, -112.6254) ccw projected
  arc A282 (-124.6393, -113.0815) -> (-123.946, -113.4931) centre (-101.8395, -75.4579) ccw projected
  arc A283 (-123.946, -113.4931) -> (-123.256, -113.3581) centre (-123.678, -113.0319) ccw projected
  arc A284 (-122.7376, -112.8461) -> (-123.256, -113.3581) centre (-121.0892, -115.0333) ccw projected
  arc A285 (-120.4477, -114.0369) -> (-122.7376, -112.8461) centre (-121.8769, -113.9881) ccw projected
  arc A286 (-120.5693, -114.7554) -> (-120.4477, -114.0369) centre (-123.185, -113.9434) ccw projected
  arc A287 (-120.5693, -114.7554) -> (-120.2835, -115.3977) centre (-120.0598, -114.9135) ccw projected
  arc A288 (-120.2835, -115.3977) -> (-119.5484, -115.729) centre (-101.8395, -75.4579) ccw projected
  arc A289 (-119.5484, -115.729) -> (-118.8779, -115.5177) centre (-119.3337, -115.2408) ccw projected
  arc A290 (-118.4201, -114.9508) -> (-118.8779, -115.5177) centre (-116.5372, -116.9398) ccw projected
  arc A291 (-116.0113, -115.8778) -> (-118.4201, -114.9508) centre (-117.4369, -115.9893) ccw projected
  arc A292 (-116.0516, -116.6053) -> (-116.0113, -115.8778) centre (-118.7417, -116.0914) ccw projected
  arc A293 (-116.0516, -116.6053) -> (-115.6957, -117.2117) centre (-115.5277, -116.7054) ccw projected
  arc A294 (-115.6957, -117.2117) -> (-114.9282, -117.4586) centre (-101.8395, -75.4579) ccw projected
  arc A295 (-114.9282, -117.4586) -> (-114.2855, -117.1735) centre (-114.7695, -116.9493) ccw projected
  arc A296 (-113.894, -116.5589) -> (-114.2855, -117.1735) centre (-111.8002, -118.3245) ccw projected
  arc A297 (-111.3966, -117.2104) -> (-113.894, -116.5589) centre (-112.8008, -117.4808) ccw projected
  arc A298 (-111.3552, -117.9379) -> (-111.3966, -117.2104) centre (-114.086, -117.7283) ccw projected
  arc A299 (-111.3552, -117.9379) -> (-110.9336, -118.5005) centre (-110.8233, -117.9787) ccw projected
  arc A300 (-110.9336, -118.5005) -> (-110.1433, -118.66) centre (-101.8395, -75.4579) ccw projected
  arc A301 (-110.1433, -118.66) -> (-109.5365, -118.3047) centre (-110.0426, -118.1361) ccw projected
  arc A302 (-109.2163, -117.6502) -> (-109.5365, -118.3047) centre (-106.9381, -119.1703) ccw projected
  arc A303 (-106.6617, -118.0179) -> (-109.2163, -117.6502) centre (-108.0268, -118.4439) ccw projected
  arc A304 (-106.5391, -118.7362) -> (-106.6617, -118.0179) centre (-109.2762, -118.8337) ccw projected
  arc A305 (-106.5391, -118.7362) -> (-106.0572, -119.2481) centre (-106.006, -118.7172) ccw projected
  arc A306 (-106.0572, -119.2481) -> (-105.254, -119.318) centre (-101.8395, -75.4579) ccw projected
  arc A307 (-105.254, -119.318) -> (-104.6908, -118.8971) centre (-105.2126, -118.7862) ccw projected
  arc A308 (-104.4459, -118.2108) -> (-104.6908, -118.8971) centre (-102.0118, -119.4663) ccw projected
  arc A309 (-101.8662, -118.2902) -> (-104.4459, -118.2108) centre (-103.175, -118.8663) ccw projected
  arc A310 (-101.6639, -118.9902) -> (-101.8662, -118.2902) centre (-104.3729, -119.3936) ccw projected
  arc A311 (-101.6639, -118.9902) -> (-101.1277, -119.445) centre (-101.1363, -118.9117) ccw projected
  arc A312 (-101.1277, -119.445) -> (-100.3217, -119.4246) centre (-101.8395, -75.4579) ccw projected
  arc A313 (-100.3217, -119.4246) -> (-99.8092, -118.9432) centre (-100.3401, -118.8915) ccw projected
  arc A314 (-99.6427, -118.2338) -> (-99.8092, -118.9432) centre (-97.0833, -119.2088) ccw projected
  arc A315 (-97.0703, -118.0239) -> (-99.6427, -118.2338) centre (-98.3064, -118.7429) ccw projected
  arc A316 (-96.791, -118.6968) -> (-97.0703, -118.0239) centre (-99.4377, -119.401) ccw projected
  arc A317 (-96.791, -118.6968) -> (-96.2072, -119.0887) centre (-96.2755, -118.5597) ccw projected
  arc A318 (-96.2072, -119.0887) -> (-95.4086, -118.9782) centre (-101.8395, -75.4579) ccw projected
  arc A319 (-95.4086, -118.9782) -> (-94.9532, -118.4425) centre (-95.4866, -118.4505) ccw projected
  arc A320 (-94.8672, -117.7189) -> (-94.9532, -118.4425) centre (-92.2147, -118.4012) ccw projected
  arc A321 (-92.3344, -117.2222) -> (-94.8672, -117.7189) centre (-93.4822, -118.0752) ccw projected
  arc A322 (-91.9815, -117.8597) -> (-92.3344, -117.2222) centre (-94.5328, -118.8558) ccw projected
  arc A323 (-91.9815, -117.8597) -> (-91.3575, -118.1837) centre (-91.4846, -117.6657) ccw projected
  arc A324 (-91.3575, -118.1837) -> (-90.5763, -117.9845) centre (-101.8395, -75.4579) ccw projected
  arc A325 (-90.5763, -117.9845) -> (-90.1838, -117.4012) centre (-90.7129, -117.4689) ccw projected
  arc A326 (-90.1793, -116.6725) -> (-90.1838, -117.4012) centre (-87.4671, -117.0535) ccw projected
  arc A327 (-87.7181, -115.8954) -> (-90.1793, -116.6725) centre (-88.7632, -116.8715) ccw projected
  arc A328 (-87.296, -116.4893) -> (-87.7181, -115.8954) centre (-89.7197, -117.7648) ccw projected
  arc A329 (-87.296, -116.4893) -> (-86.6397, -116.7415) centre (-86.824, -116.2409) ccw projected
  arc A330 (-86.6397, -116.7415) -> (-85.8857, -116.456) centre (-101.8395, -75.4579) ccw projected
  arc A331 (-85.8857, -116.456) -> (-85.5609, -115.8324) centre (-86.0791, -115.9589) ccw projected
  arc A332 (-85.638, -115.1078) -> (-85.5609, -115.8324) centre (-82.9002, -115.1828) ccw projected
  arc A333 (-83.2793, -114.06) -> (-85.638, -115.1078) centre (-84.2086, -115.147) ccw projected
  arc A334 (-82.7934, -114.603) -> (-83.2793, -114.06) centre (-85.059, -116.1418) ccw projected
  arc A335 (-82.7934, -114.603) -> (-82.1129, -114.78) centre (-82.3521, -114.3033) ccw projected
  arc A336 (-82.1129, -114.78) -> (-81.3956, -114.4119) centre (-101.8395, -75.4579) ccw projected
  arc A337 (-81.3956, -114.4119) -> (-81.1428, -113.7559) centre (-81.6435, -113.9396) ccw projected
  arc A338 (-81.3005, -113.0445) -> (-81.1428, -113.7559) centre (-78.5716, -112.8125) ccw projected
  arc A339 (-79.074, -111.7392) -> (-81.3005, -113.0445) centre (-79.8756, -112.9234) ccw projected
  arc A340 (-78.5303, -112.2243) -> (-79.074, -111.7392) centre (-80.6094, -114.0072) ccw projected
  arc A341 (-78.5303, -112.2243) -> (-77.8343, -112.3241) centre (-78.1254, -111.8771) ccw projected
  arc A342 (-77.8343, -112.3241) -> (-77.1627, -111.878) centre (-101.8395, -75.4579) ccw projected
  arc A343 (-77.1627, -111.878) -> (-76.9849, -111.1978) centre (-77.4619, -111.4364) ccw projected
  arc A344 (-77.2213, -110.5086) -> (-76.9849, -111.1978) centre (-74.5355, -109.9724) ccw projected
  arc A345 (-75.1549, -108.9621) -> (-77.2213, -110.5086) centre (-75.819, -110.2286) ccw projected
  arc A346 (-74.5603, -109.3834) -> (-75.1549, -108.9621) centre (-76.4267, -111.3877) ccw projected
  arc A347 (-74.5603, -109.3834) -> (-73.8575, -109.4046) centre (-74.1968, -108.993) ccw projected
  arc A348 (-73.8575, -109.4046) -> (-73.2401, -108.8861) centre (-101.8395, -75.4579) ccw projected
  arc A349 (-73.2401, -108.8861) -> (-73.1396, -108.1902) centre (-73.5869, -108.4808) ccw projected
  arc A350 (-73.4517, -107.5318) -> (-73.1396, -108.1902) centre (-70.8428, -106.6983) ccw projected
  arc A351 (-71.5714, -105.7637) -> (-73.4517, -107.5318) centre (-72.0895, -107.0966) ccw projected
  arc A352 (-70.9334, -106.1157) -> (-71.5714, -105.7637) centre (-72.5637, -108.3165) ccw projected
  arc A353 (-70.9334, -106.1157) -> (-70.2327, -106.0581) centre (-70.6159, -105.6871) ccw projected
  arc A354 (-70.2327, -106.0581) -> (-69.6772, -105.4738) centre (-101.8395, -75.4579) ccw projected
  arc A355 (-69.6772, -105.4738) -> (-69.6552, -104.771) centre (-70.0672, -105.1098) ccw projected
  arc A356 (-70.039, -104.1517) -> (-69.6552, -104.771) centre (-67.5398, -103.0314) ccw projected
  arc A357 (-68.3685, -102.1842) -> (-70.039, -104.1517) centre (-68.7341, -103.5667) ccw projected
  arc A358 (-67.6951, -102.4626) -> (-68.3685, -102.1842) centre (-69.0688, -104.832) ccw projected
  arc A359 (-67.6951, -102.4626) -> (-67.0053, -102.3269) centre (-67.4276, -102.0011) ccw projected
  arc A360 (-67.0053, -102.3269) -> (-66.5187, -101.684) centre (-101.8395, -75.4579) ccw projected
  arc A361 (-66.5187, -101.684) -> (-66.5755, -100.9832) centre (-66.947, -101.366) ccw projected
  arc A362 (-67.0263, -100.4107) -> (-66.5755, -100.9832) centre (-64.6683, -99.0176) ccw projected
  arc A363 (-65.5866, -98.2686) -> (-67.0263, -100.4107) centre (-65.7951, -99.6834) ccw projected
  arc A364 (-64.8863, -98.4698) -> (-65.5866, -98.2686) centre (-65.986, -100.9782) ccw projected
  arc A365 (-64.8863, -98.4698) -> (-64.2159, -98.2577) centre (-64.6721, -97.9813) ccw projected
  arc A366 (-64.2159, -98.2577) -> (-63.8044, -97.5644) centre (-101.8395, -75.4579) ccw projected
  arc A367 (-63.8044, -97.5644) -> (-63.9393, -96.8744) centre (-64.2656, -97.2964) ccw projected
  arc A368 (-64.4514, -96.356) -> (-63.9393, -96.8744) centre (-62.2642, -94.7076) ccw projected
  arc A369 (-63.2606, -94.0662) -> (-64.4514, -96.356) centre (-63.3094, -95.4953) ccw projected
  arc A370 (-62.5421, -94.1877) -> (-63.2606, -94.0662) centre (-63.354, -96.8034) ccw projected
  arc A371 (-62.5421, -94.1877) -> (-61.8997, -93.9019) centre (-62.384, -93.6782) ccw projected
  arc A372 (-61.8997, -93.9019) -> (-61.5684, -93.1668) centre (-101.8395, -75.4579) ccw projected
  arc A373 (-61.5684, -93.1668) -> (-61.7798, -92.4963) centre (-62.0567, -92.9521) ccw projected
  arc A374 (-62.3466, -92.0385) -> (-61.7798, -92.4963) centre (-60.3577, -90.1556) ccw projected
  arc A375 (-61.4197, -89.6297) -> (-62.3466, -92.0385) centre (-61.3082, -91.0553) ccw projected
  arc A376 (-60.6921, -89.67) -> (-61.4197, -89.6297) centre (-61.2061, -92.3602) ccw projected
  arc A377 (-60.6921, -89.67) -> (-60.0858, -89.3141) centre (-60.5921, -89.1461) ccw projected
  arc A378 (-60.0858, -89.3141) -> (-59.8389, -88.5466) centre (-101.8395, -75.4579) ccw projected
  arc A379 (-59.8389, -88.5466) -> (-60.124, -87.9039) centre (-60.3481, -88.3879) ccw projected
  arc A380 (-60.7385, -87.5124) -> (-60.124, -87.9039) centre (-58.9729, -85.4187) ccw projected
  arc A381 (-60.0871, -85.015) -> (-60.7385, -87.5124) centre (-59.8167, -86.4192) ccw projected
  arc A382 (-59.3596, -84.9736) -> (-60.0871, -85.015) centre (-59.5691, -87.7044) ccw projected
  arc A383 (-59.3596, -84.9736) -> (-58.7969, -84.552) centre (-59.3188, -84.4417) ccw projected
  arc A384 (-58.7969, -84.552) -> (-58.6375, -83.7617) centre (-101.8395, -75.4579) ccw projected
  arc A385 (-58.6375, -83.7617) -> (-58.9928, -83.1549) centre (-59.1613, -83.661) ccw projected
  arc A386 (-59.6473, -82.8348) -> (-58.9928, -83.1549) centre (-58.1272, -80.5565) ccw projected
  arc A387 (-59.2796, -80.2801) -> (-59.6473, -82.8348) centre (-58.8536, -81.6452) ccw projected
  arc A388 (-58.5613, -80.1575) -> (-59.2796, -80.2801) centre (-58.4638, -82.8946) ccw projected
  arc A389 (-58.5613, -80.1575) -> (-58.0494, -79.6756) centre (-58.5803, -79.6244) ccw projected
  arc A390 (-58.0494, -79.6756) -> (-57.9794, -78.8724) centre (-101.8395, -75.4579) ccw projected
  arc A391 (-57.9794, -78.8724) -> (-58.4004, -78.3092) centre (-58.5112, -78.831) ccw projected
  arc A392 (-59.0867, -78.0643) -> (-58.4004, -78.3092) centre (-57.8312, -75.6302) ccw projected